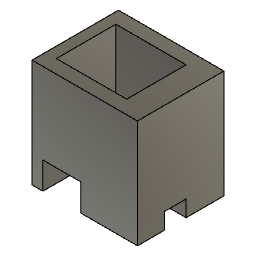
Switch Mount v0 (Autodesk Fusion 360 design; units mm, degrees)
Autodesk Fusion 360 part; units mm, degrees
sketch "Sketch1" plane through (0, 0, 0) normal (0, 0, 1) x (1, 0, 0)
  line L0 (0, 0) -> (19.5, 0)
  line L1 (19.5, 0) -> (19.5, 16)
  line L2 (19.5, 16) -> (0, 16)
  line L3 (0, 16) -> (0, 0)
  dimension "d1" = 19.5
  dimension "d2" = 16
  constraint horizontal L0
  constraint vertical L1
  constraint horizontal L2
  constraint vertical L3
  constraint coincident L0.start L3.end
  measures "d1" distance of L0.start L0.end
  measures "d2" distance of L0.start L2.end
extrude "Extrude1" add sketch "Sketch1" along normal blind 20
sketch "Sketch2" plane through (0, 0, 0) normal (0, -1, 0) x (1, 0, 0)
  line L0 (0, 0) -> (19.5, 0)
  line L1 (19.5, 0) -> (19.5, 20)
  line L2 (19.5, 20) -> (0, 20)
  line L3 (0, 20) -> (0, 0)
  line L4 (2, 0) -> (9, 0)
  line L5 (9, 0) -> (9, 5)
  line L6 (9, 5) -> (2, 5)
  line L7 (2, 5) -> (2, 0)
  dimension "d5" = 2
  constraint horizontal L4
  constraint vertical L5
  constraint horizontal L6
  constraint vertical L7
  constraint coincident L0 L4.start
  measures "d5" distance of L3 L7
extrude "Extrude2" cut sketch "Sketch2" against normal blind 47 contours L0 L4 L5 L6 L7
sketch "Sketch3" plane through (0, 0, 20) normal (0, 0, 1) x (-1, 0, 0)
  line L0 (0, -16) -> (0, 0)
  line L1 (0, 0) -> (-19.5, 0)
  line L2 (-19.5, 0) -> (-19.5, -16)
  line L3 (-19.5, -16) -> (0, -16)
  line L4 (5, -8) -> (-24, -8) construction
  line L5 (-2, -13.5) -> (-15, -13.5)
  line L6 (-15, -13.5) -> (-15, -2.5)
  line L7 (-15, -2.5) -> (-2, -2.5)
  line L8 (-2, -2.5) -> (-2, -13.5)
  dimension "d8" = 8
  dimension "d9" = 13
  dimension "d10" = 11
  dimension "d11" = 2
  dimension "d12" = 5.5
  constraint perpendicular L2 L4
  constraint horizontal L5
  constraint vertical L6
  constraint horizontal L7
  constraint vertical L8
  measures "d8" distance of L3 L4
  measures "d9" distance of L5.start L5.end
  measures "d10" distance of L5.start L7.end
  measures "d11" distance of L0 L8
  measures "d12" distance of L4 L5
extrude "Extrude3" cut sketch "Sketch3" against normal blind 36 contours L5 L6 L7 L8
sketch "Sketch4" plane through (19.5, 0, 0) normal (1, 0, 0) x (0, 1, 0)
  line L0 (0, 0) -> (16, 0)
  line L1 (16, 0) -> (16, 20)
  line L2 (16, 20) -> (0, 20)
  line L3 (0, 20) -> (0, 0)
  line L4 (5, 0) -> (9, 0)
  line L5 (9, 0) -> (9, 3)
  line L6 (9, 3) -> (5, 3)
  line L7 (5, 3) -> (5, 0)
  constraint horizontal L4
  constraint vertical L5
  constraint horizontal L6
  constraint vertical L7
  constraint coincident L0 L4.start
extrude "Extrude4" cut sketch "Sketch4" against normal blind 8 contours L0 L4 L5 L6 L7
